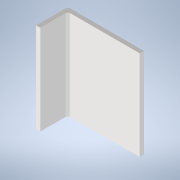
# Autodesk Inventor part: stativ
Saved by Autodesk Inventor 2022 (Build 260153000, 153)
## iProperties
Created: 2022-01-02
Part Number: stativ
Material: Generisch
Document SubType Name: Modeling
Designer: Jan
Density: 1 g/cm^3
Appearance: Vorgabe
Author: Jan
Autodesk Inventor part; units mm, degrees
ref_plane "YZ Plane" through (0, 0, 0) normal (1, 0, 0) x (0, 1, 0)
ref_plane "XZ Plane" through (0, 0, 0) normal (0, 1, 0) x (-1, 0, 0)
ref_plane "XY Plane" through (0, 0, 0) normal (0, 0, 1) x (1, 0, 0)
sketch "Skizze1" plane through (0, 0, 0) normal (0, 0, 1) x (1, 0, 0)
  line L0 (0, 10) -> (50, 10)
  line L1 (50, 10) -> (50, -45)
  line L2 (50, -45) -> (0, -45)
  line L3 (0, -45) -> (-5, -45)
  line L4 (-5, -45) -> (-5, 10)
  line L5 (-5, 10) -> (0, 10)
  point P0 (0, 0)
  dimension "d0" = 10
  dimension "d1" = 50
  dimension "d2" = 55
  dimension "d3" = 50
  dimension "d6" = 5
  constraints: 12 end point, 4 perpendicular, 2 horizontal
  measures "d0" distance of L0.start point (0, 0)
  measures "d1" distance of L0.start L0.end
  measures "d2" distance of L0.end L1.end
  measures "d3" distance of L1.end L2.end
  measures "d6" distance of L2.end L3.end
extrude "Extrusion1" add sketch "Skizze1" along normal blind 3
sketch "Skizze3" plane through (0, 0, 3) normal (0, 0, 1) x (1, 0, 0)
  line L0 (50, 10) -> (-5, 10) projected
  line L1 (-5, 10) -> (-5, -45) projected
  line L2 (-5, 10) -> (-2, 10)
  line L3 (-2, 10) -> (-2, -45)
  line L4 (-5, -45) -> (50, -45) projected
  line L5 (-5, -45) -> (-5, 10)
  point P0 (0, 0)
  dimension "d13" = 3
  constraints: 6 end point, 2 point on line, 1 parallel, 1 perpendicular
  measures "d13" distance of L0.end L2.end
extrude "Extrusion3" add sketch "Skizze3" along normal blind 20
fillet "Rundung2" radius 2 2 edges at (-2, -17.5, 3) (-5, -17.5, 0)
sketch "Skizze4" plane through (0, 0, 3) normal (0, 0, 1) x (1, 0, 0)
  circle A0 centre (46, -36.5) radius 3 projected
  circle A1 centre (4, 6) radius 3 projected
  circle A2 centre (4, 6) radius 1.8 projected
  circle A3 centre (46, -36.5) radius 1.8 projected
  point P0 (0, 0)
  dimension "d17" = 3.6
  dimension "d18" = 6
  constraints: 1 coincident
  measures "d17" diameter of A2
  measures "d18" diameter of A1
hole "Bohrung1" at (4, 6, 3) at (46, -36.5, 3) direction (0, 0, -1) diameter 6 end through all counterbore diameter 7 counterbore depth 1
